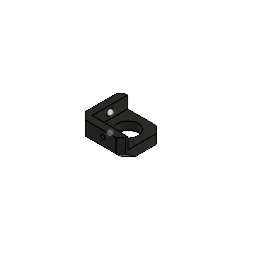
Bed Corner Support (Autodesk Fusion 360 design; units mm, degrees)
Autodesk Fusion 360 part; units mm, degrees
sketch "Sketch3" plane through (-5, 0, 0) normal (1, 0, 0) x (0, 1, 0)
  line L0 (17, 36) -> (47, 36)
  line L1 (47, 36) -> (47, 46)
  line L2 (47, 46) -> (17, 46)
  line L3 (17, 46) -> (17, 36)
  line L4 (17, 46) -> (47, 36) construction
  line L5 (33.5877, 38.25) -> (35.1754, 41)
  line L6 (35.1754, 41) -> (33.5877, 43.75)
  line L7 (33.5877, 43.75) -> (30.4123, 43.75)
  line L8 (30.4123, 43.75) -> (28.8246, 41)
  line L9 (28.8246, 41) -> (30.4123, 38.25)
  line L10 (30.4123, 38.25) -> (33.5877, 38.25)
  point P0 (32, 41)
  dimension "d1" = 5.5
  constraint coincident L2.end L3.start
  constraint coincident L0.end L1.start
  constraint midpoint L4 P0
  constraint horizontal L10
  measures "d1" distance of L7 L10
sketch "Sketch4" plane through (0, 17, 0) normal (0, 1, 0) x (-1, 0, 0)
  line L0 (-25, 36) -> (5, 36)
  line L1 (5, 36) -> (5, 46)
  line L2 (5, 46) -> (-25, 46)
  line L3 (-25, 46) -> (-25, 36)
  line L4 (5, 46) -> (-25, 36) construction
  line L5 (-6.8246, 41) -> (-8.4123, 43.75)
  line L6 (-8.4123, 43.75) -> (-11.5877, 43.75)
  line L7 (-11.5877, 43.75) -> (-13.1754, 41)
  line L8 (-13.1754, 41) -> (-11.5877, 38.25)
  line L9 (-11.5877, 38.25) -> (-8.4123, 38.25)
  line L10 (-8.4123, 38.25) -> (-6.8246, 41)
  point P0 (-10, 41)
  dimension "d2" = 5.5
  constraint coincident L1.end L2.start
  constraint coincident L0.start L3.end
  constraint midpoint L4 P0
  constraint horizontal L9
  measures "d2" distance of L6 L9
sketch "Sketch1" plane through (0, 0, 28) normal (0, 0, 1) x (-1, 0, 0)
  line L0 (5, -47) -> (-25, -47)
  line L1 (-25, -47) -> (-25, -17)
  line L2 (-25, -17) -> (5, -17)
  line L3 (5, -17) -> (5, -47)
  line L4 (-25, -17) -> (5, -47) construction
  line L5 (5, -47) -> (11, -47)
  line L6 (11, -47) -> (11, -11)
  line L7 (11, -11) -> (-25, -11)
  line L8 (-25, -11) -> (-25, -17)
  circle A0 centre (-10, -32) radius 2.75
  circle A1 centre (-10, -32) radius 7.5 construction
  circle A2 centre (-10, -32) radius 8
  dimension "d750" = 30
  dimension "d751" = 30
  dimension "d758" = 6
  dimension "d759" = 6
  dimension "d805" = 0
  dimension "d806" = 0
  dimension "d807" = 0
  dimension "d808" = 0
  dimension "d905" = 0
  dimension "d906" = 0
  dimension "d907" = 0
  dimension "d908" = 0
  dimension "d917" = 0
  dimension "d918" = 0
  dimension "d919" = 0
  dimension "d920" = 0
  dimension "d988" = 0
  dimension "d989" = 0
  dimension "d990" = 0
  dimension "d991" = 0
  dimension "d1049" = 0
  dimension "d1050" = 0
  dimension "d1051" = 0
  dimension "d1052" = 0
  dimension "d1061" = 0
  dimension "d1062" = 0
  dimension "d1063" = 0
  dimension "d1064" = 0
  dimension "d1243" = 0
  dimension "d1244" = 0
  dimension "d1245" = 0
  dimension "d1246" = 0
  dimension "d1299" = 0
  dimension "d1300" = 0
  dimension "d1301" = 0
  dimension "d1302" = 0
  dimension "d1319" = 0
  dimension "d1320" = 0
  dimension "d1321" = 0
  dimension "d1322" = 0
  dimension "d1364" = 0
  dimension "d1365" = 0
  dimension "d1366" = 0
  dimension "d1367" = 0
  constraint horizontal L0
  constraint vertical L1
  constraint horizontal L2
  constraint vertical L3
  constraint perpendicular L3 L5
  constraint perpendicular L5 L6
  constraint perpendicular L1 L7
  constraint perpendicular L2 L8
  constraint midpoint L4 A0.centre
  measures "d750" distance of L0.start L0.end
  measures "d751" distance of L0.start L2.end
  measures "d758" distance of L1.end L7.end
  measures "d759" distance of L0.start L5.end
extrude "Extrude1" add sketch "Sketch1" along normal blind 8 contours L0 L1 L2 L3 | L2 L3 L5 L6 L7 L8
chamfer "Chamfer3" distance 2 angle 40 1 edges at (17.4586, 29.1071, 28) measured on face at (2.0398, 32.7965, 30.6667)
move_face "OffsetFaces1" offset -0.5 1 faces at (2.0398, 32.7965, 32)
extrude "Extrude2" add sketch "Sketch1" along normal blind 18 contours L2 L3 L5 L6 L7 L8
extrude "Extrude4" cut sketch "Sketch4" against normal blind 3 contours L5 L6 L7 L8 L9 L10
extrude "Extrude5" cut sketch "Sketch3" against normal blind 3 contours L5 L6 L7 L8 L9 L10
hole "Hole5" at (10, 17, 41) direction (0, -1, 0) diameter 3.5 depth 10 tip angle 118
hole "Hole6" at (-5, 32, 41) direction (-1, 0, 0) diameter 3.5 depth 10 tip angle 118
chamfer "Chamfer2" distance 4 angle 45 2 edges at (25, 11, 37) (-11, 47, 37)
chamfer "Chamfer4" distance 6 angle 45 2 edges at (-11, 11, 37) (25, 47, 32)
chamfer "Chamfer1" distance 6 angle 45 5 edges at (8, 11, 28) (-11, 30, 28) (23, 13, 28) (-9, 45, 28) (-8, 14, 28)
equation "d751 = d750"
equation "d759 = d758"
named bodies: "Bed Corner Support"
